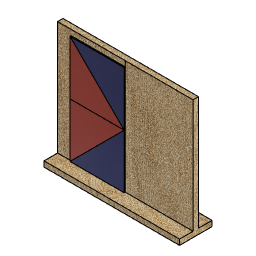
Evolution Door (Autodesk Fusion 360 design; units mm, degrees)
Autodesk Fusion 360 part; units mm, degrees
note: some values were not read from the file. Set by a fixed rule: which sketch regions a step uses.
sketch "Base" plane through (0, 0, 0) normal (0, 0, 1) x (1, 0, 0) in component "Doorframe"
  line L0 (125, -30) -> (-125, -30)
  line L1 (-125, -30) -> (-125, 30)
  line L2 (-125, 30) -> (125, 30)
  line L3 (125, 30) -> (125, -30)
  line L4 (125, -30) -> (-125, 30) construction
  line L5 (-125, -30) -> (125, 30) construction
  line L6 (-100, 4.6686) -> (-100, -5.0109)
  line L7 (-125, -5.3314) -> (-125, 4.6686)
  line L8 (125, 5) -> (0, 5)
  line L9 (0, 5) -> (0, -5)
  line L10 (0, -5) -> (125, -5)
  line L11 (125, -5) -> (125, 5)
  line L12 (-125, 4.9891) -> (-100, 4.9891)
  line L13 (-100, 4.9891) -> (-100, -5.0109)
  line L14 (-100, -5.0109) -> (-125, -5.0109)
  line L15 (-125, -5.0109) -> (-125, 4.9891)
  dimension "d1" = 250
  dimension "d2" = 60
  dimension "d3" = 25
  dimension "d4" = 10
  dimension "d5" = 125
  dimension "d31" = 10
  constraint horizontal L0
  constraint perpendicular L0 L1
  constraint parallel L0 L2
  constraint parallel L1 L3
  constraint coincident L4 origin
  constraint coincident L5 origin
  constraint vertical L6
  constraint vertical L7
  constraint coincident L1 L7.end
  constraint horizontal L8
  constraint vertical L9
  constraint horizontal L10
  constraint vertical L11
  constraint coincident L3 L8.start
  constraint horizontal L12
  constraint vertical L13
  constraint horizontal L14
  constraint vertical L15
  constraint coincident L1 L12.start
  measures "d1" distance of L1.end L2.end
  measures "d2" distance of L0.end L1.end
  measures "d3" distance of L7.end L6.start
  measures "d4" distance of L7.end L7.start
  measures "d5" distance of L8.start L8.end
  measures "d31" distance of L12.start L14.end
extrude "Extrude1" add sketch "Base" along normal blind 220 contours L3 L8 L9 L10 L11 | L1 L6 L7 L12 L13 L14 L15 makes body 1 at (-116.6667, 4.9891, 73.3333) makes body 2 at (41.6667, -5, 73.3333) in component "Doorframe"
extrude "Extrude2" add sketch "Base" along normal blind 10 contours L0 L1 L2 L3 L6 L7 L8 L9 L10 L12 L13 L14 bodies 1 2 in component "Doorframe"
sketch "lower half bottom" plane through (0, 0, 0) normal (0, 1, 0) x (1, 0, 0) in component "Lower half bottom"
  line L0 (0, -10) -> (0, -110)
  line L1 (0, -110) -> (-100, -10)
  line L2 (-100, -10) -> (0, -10)
  dimension "d10" = 100
  constraint vertical L0
  constraint perpendicular L0 L2
  measures "d10" distance of L0.start L0.end
sketch "lower half top" plane through (0, 0, 0) normal (0, 1, 0) x (1, 0, 0) in component "Lower half top"
  line L0 (-100, -10) -> (-100, -110)
  line L1 (-100, -110) -> (0, -110)
  line L2 (0, -110) -> (-100, -10)
  constraint vertical L0
  constraint perpendicular L0 L1
sketch "upper half bottom" plane through (0, 0, 0) normal (0, 1, 0) x (1, 0, 0) in component "Upper half bottom"
  line L0 (-100, -110) -> (-100, -210)
  line L1 (-100, -210) -> (0, -110)
  line L2 (0, -110) -> (-100, -110)
  dimension "d11" = 100
  constraint vertical L0
  constraint perpendicular L0 L2
  measures "d11" distance of L0.start L0.end
sketch "upper half top" plane through (0, 0, 0) normal (0, 1, 0) x (1, 0, 0) in component "Upper half top"
  line L0 (0, -110) -> (0, -210)
  line L1 (0, -210) -> (-100, -210)
  line L2 (-100, -210) -> (0, -110)
  constraint vertical L0
  constraint perpendicular L0 L1
extrude "Extrude1'" add sketch "upper half top" along normal blind -5 and the other way blind 7 separate body makes body 3 in component "Upper half top"
extrude "Extrude1''" add sketch "upper half bottom" along normal blind -5 and the other way blind 7 separate body makes body 4 in component "Upper half bottom"
extrude "Extrude1'''" add sketch "lower half top" along normal blind -5 and the other way blind 7 separate body makes body 5 in component "Lower half top"
extrude "Extrude1''''" add sketch "lower half bottom" along normal blind -5 and the other way blind 7 separate body makes body 6 in component "Lower half bottom"
sketch "Upper frame" plane through (-100, 0, 0) normal (1, 0, 0) x (0, 1, 0) in component "Doorframe"
  line L0 (-5.0109, 10) -> (4.9891, 10)
  line L1 (4.9891, 220) -> (-5.0109, 220)
  line L2 (4.9891, 10) -> (4.9891, 220)
  line L3 (-5.0109, 220) -> (-5.0109, 10)
  line L4 (-5.0109, 220) -> (4.9891, 220)
  line L5 (4.9891, 220) -> (4.9891, 210)
  line L6 (4.9891, 210) -> (-5.0109, 210)
  line L7 (-5.0109, 210) -> (-5.0109, 220)
  dimension "d32" = 10
  dimension "d33" = 10
  constraint horizontal L4
  constraint vertical L5
  constraint horizontal L6
  constraint vertical L7
  constraint coincident L1.end L3.start
  measures "d32" distance of L1.end L1.start
  measures "d33" distance of L1.end L6.end
extrude "Extrude3" add sketch "Upper frame" along normal blind 100 contours L1 L2 L3 L4 L5 L6 L7 bodies 1 in component "Doorframe"
component "Doorframe" placed x (1, 0, 0) y (0, 1, 0) z (0, 0, 1) at (0, 0, 0)
component "Lower half bottom" placed x (1, 0, 0) y (0, 1, 0) z (0, 0, 1) at (0, 0, 0)
component "Lower half top" placed x (1, 0, 0) y (0, 1, 0) z (0, 0, 1) at (0, 0, 0)
component "Upper half bottom" placed x (1, 0, 0) y (0, 1, 0) z (0, 0, 1) at (0, 0, 0)
component "Upper half top" placed x (1, 0, 0) y (0, 1, 0) z (0, 0, 1) at (0, 0, 0)
named bodies: "Doorframe", "Upper half top", "Upper half bottom", "Lower half top", "Lower half bottom"
